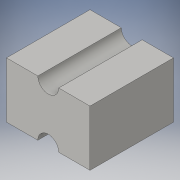
# Autodesk Inventor part: MiddleOfSquareSupport
Saved by Autodesk Inventor 2016 SP1 (Build 200210100, 210)
## iProperties
Created: 2015-12-08
Part Number: MiddleOfSquareSupport
Material: Generic
Document SubType Name: Modeling
Designer: steele
Density: 1 g/cm^3
Appearance: Default
Author: steele
Autodesk Inventor part; units mm, degrees
ref_plane "YZ Plane" through (0, 0, 0) normal (1, 0, 0) x (0, 1, 0)
ref_plane "XZ Plane" through (0, 0, 0) normal (0, 1, 0) x (-1, 0, 0)
ref_plane "XY Plane" through (0, 0, 0) normal (0, 0, 1) x (1, 0, 0)
sketch "Sketch1" plane through (0, 0, 0) normal (0, 1, 0) x (-1, 0, 0)
  line L0 (-19.05, 19.05) -> (-19.05, -19.05)
  line L1 (-19.05, -19.05) -> (19.05, -19.05)
  line L2 (19.05, -19.05) -> (19.05, 19.05)
  line L3 (19.05, 19.05) -> (-19.05, 19.05)
  line L4 (-19.05, 19.05) -> (19.05, -19.05) construction
  line L5 (-19.05, -19.05) -> (19.05, 19.05) construction
  point P0 (0, 0)
  dimension "d4" = 38.1
  constraints: 12 end point, 2 midpoint, 2 parallel, 2 perpendicular, 1 vertical
  measures "d4" distance of L0.start L0.end
extrude "Extrusion1" add sketch "Sketch1" along normal blind 25.4
sketch "Sketch3" plane through (-19.05, 0, 19.05) normal (0, 0, 1) x (1, 0, 0)
  line L0 (38.1, 25.4) -> (0, 25.4) construction
  point P0 (19.05, 0)
  point P1 (19.05, 25.4)
  point P2 (19.05, 0)
  constraints: 1 coincident, 1 midpoint
hole "Hole1" at (0, 25.4, 19.05) at (0, 0, 19.05) direction (0, 0, -1) diameter 9.525 end through all
equation "\"d4\" = width"
equation "\"d6\" = deltaBottomToTop"
equation "\"d9\" = bottomHoleDiam"
equation "\"bottomHoleDiam\" = 9.525"
equation "\"width\" = 38.1"
equation "\"deltaBottomToTop\" = 25.4"
equation "\"d0\" = width"
equation "\"d1\" = heightOfBottomHole"
equation "\"d2\" = 0"
equation "\"d3\" = bottomHoleDiam"
equation "\"d5\" = 0"
equation "\"height\" = deltaBottomToTop + heightOfBottomHole + heightOfTopHole"
equation "\"heightOfBottomHole\" = 11.1125"
equation "\"heightOfTopHole\" = 11.1125"
body "Solid1"
